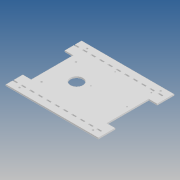
# Autodesk Inventor part: 000.101 - Bottom
Saved by Autodesk Inventor 2020 (Build 240168000, 168)
## iProperties
Created: 2021-06-27
Part Number: 000.101 - Bottom
Material: Типовые
Document SubType Name: Modeling
Designer: Петров Иван
Mass: 102.402 g
Surface Area: 732.006 cm^2
Volume: 102.402 cm^3
Density: 1 g/cm^3
Appearance: По умолчанию
Author: Петров Иван
Autodesk Inventor part; units mm, degrees
ref_plane "YZ Plane" through (0, 0, 0) normal (1, 0, 0) x (0, 1, 0)
ref_plane "XZ Plane" through (0, 0, 0) normal (0, 1, 0) x (-1, 0, 0)
ref_plane "XY Plane" through (0, 0, 0) normal (0, 0, 1) x (1, 0, 0)
sketch "Эскиз9" plane through (0, 0, 0) normal (0, 1, 0) x (-1, 0, 0)
  line L0 (-110, 90) -> (110, 90)
  line L1 (110, 90) -> (110, -90)
  line L2 (110, -90) -> (-110, -90)
  line L3 (-110, -90) -> (-110, 90)
  line L4 (-110, 90) -> (110, -90) construction
  line L5 (110, 90) -> (-110, -90) construction
  point P0 (0, 0)
  dimension "d50" = 220
  dimension "d51" = 180
  constraints: 12 end point, 2 midpoint, 2 parallel, 1 horizontal, 1 perpendicular
  measures "d50" distance of L1.end L2.end
  measures "d51" distance of L0.end L1.end
extrude "Выдавливание9" add sketch "Эскиз9" along normal blind 3
sketch "Эскиз10" plane through (0, 0, 0) normal (0, -1, 0) x (1, 0, 0)
  circle A0 centre (99.9996, -40) radius 2 projected
  circle A1 centre (99.9996, 0) radius 2 projected
  circle A2 centre (99.9996, 40) radius 2 projected
  circle A3 centre (-99.9997, 0) radius 2 projected
  circle A4 centre (-99.9997, -40) radius 2 projected
  circle A5 centre (-99.9997, 40) radius 2 projected
  point P0 (0, 0)
extrude "Выдавливание10" cut sketch "Эскиз10" against normal blind 3
sketch "Эскиз11" plane through (0, 3, 0) normal (0, 1, 0) x (1, 0, 0)
  circle A0 centre (87.4999, 80.5) radius 2 projected
  circle A1 centre (-87.5001, 80.5) radius 2 projected
  circle A2 centre (-87.5001, -80.5) radius 2 projected
  circle A3 centre (87.4999, -80.5) radius 2 projected
  point P0 (0, 0)
extrude "Выдавливание11" cut sketch "Эскиз11" against normal blind 10
sketch "Эскиз12" plane through (0, 3, 0) normal (0, 1, 0) x (1, 0, 0)
  line L0 (-110, 90) -> (-110, -90) projected
  line L1 (-110, 50) -> (-90, 50)
  line L2 (-90, 50) -> (-90, -50)
  line L3 (-90, -50) -> (-110, -50)
  line L4 (-110, -50) -> (-110, 50)
  point P0 (0, 0)
  dimension "d61" = 20
  dimension "d62" = 50
  dimension "d63" = 100
  constraints: 8 end point, 2 parallel, 1 horizontal, 1 perpendicular, 1 point on line
  measures "d61" distance between parallel lines of L0 L2
  measures "d62" distance from line of point (0, 0) L1
  measures "d63" distance of L1.end L2.end
extrude "Выдавливание12" cut sketch "Эскиз12" against normal blind 10
mirror "Зеркальное отражение1" about plane through (0, 0, 0) normal (1, 0, 0) of "Выдавливание12"
sketch "Эскиз13" plane through (0, 3, 0) normal (0, 1, 0) x (1, 0, 0)
  circle A0 centre (-31.6806, 0) radius 15
  point P0 (0, 0)
  dimension "d66" = 30
  constraints: 1 centre point
  measures "d66" diameter of A0
extrude "Выдавливание13" cut sketch "Эскиз13" against normal blind 10
sketch "Эскиз14" plane through (0, 0, 0) normal (0, -1, 0) x (1, 0, 0)
  circle A0 centre (-73, 42.4597) radius 2 projected
  circle A1 centre (-73, -39.4484) radius 2 projected
  point P0 (0, 0)
extrude "Выдавливание14" cut sketch "Эскиз14" against normal blind 10
sketch "Эскиз15" plane through (0, 0, 0) normal (0, -1, 0) x (1, 0, 0)
  circle A0 centre (-6, -8) radius 1.375 projected
  circle A1 centre (80, -8) radius 1.375 projected
  circle A2 centre (80, -66) radius 1.375 projected
  circle A3 centre (-6, -66) radius 1.375 projected
  point P0 (0, 0)
extrude "Выдавливание15" cut sketch "Эскиз15" against normal blind 10
sketch "Эскиз16" plane through (0, 3, 0) normal (0, 1, 0) x (1, 0, 0)
  line L0 (-110, -50) -> (-110, -90) projected
  line L1 (-110, -71.5) -> (-100, -71.5)
  line L2 (-100, -71.5) -> (-100, -74.5)
  line L3 (-100, -74.5) -> (-110, -74.5)
  line L4 (-110, -74.5) -> (-110, -71.5)
  circle A0 centre (-87.5001, -80.5) radius 2 projected
  point P0 (0, 0)
  dimension "d73" = 10
  dimension "d74" = 3
  dimension "d75" = 6
  constraints: 8 end point, 2 parallel, 1 horizontal, 1 perpendicular, 1 point on line
  measures "d73" distance of L2.end L3.end
  measures "d74" distance of L1.end L2.end
  measures "d75" distance from line of A0.centre L3
extrude "Выдавливание16" cut sketch "Эскиз16" against normal blind 10 contours L1 L2 L3 L0
pattern_linear "Прямоуг.массив5" count 12 spacing 20 along (1, 0, 0) of "Выдавливание16"
mirror "Зеркальное отражение2" about plane through (0, 0, 0) normal (0, 0, 1) of "Выдавливание16", "Прямоуг.массив5"
